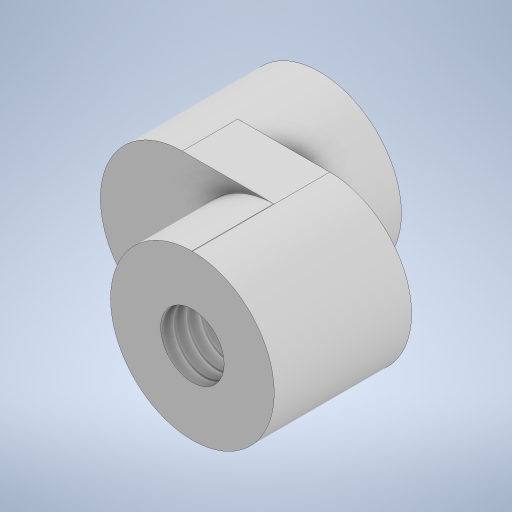
# Autodesk Inventor part: PC104_EM-113 standoff_3.57
Saved by Autodesk Inventor 2024 (Build 280153000, 153)
## iProperties
Created: 2023-04-19
Part Number: PC104_EM-113 standoff_3.57
Material: Generic
Document SubType Name: Modeling
Designer: Owner
Density: 1 g/cm^3
Appearance: Default
Author: Owner
Autodesk Inventor part; units mm, degrees
ref_plane "YZ Plane" through (0, 0, 0) normal (1, 0, 0) x (0, 1, 0)
ref_plane "XZ Plane" through (0, 0, 0) normal (0, 1, 0) x (-1, 0, 0)
ref_plane "XY Plane" through (0, 0, 0) normal (0, 0, 1) x (1, 0, 0)
sketch "Sketch2" plane through (0, 0, 0) normal (0, 0, 1) x (1, 0, 0)
  arc A0 (3.57, -3.175) -> (3.57, 3.175) centre (3.57, 0) ccw
  arc A1 (0, 3.175) -> (0, -3.175) centre (0, 0) ccw
  line L0 (0, 3.175) -> (3.57, 3.175)
  line L1 (0, -3.175) -> (3.57, -3.175)
  dimension "d14" = 6.35
  dimension "d15" = 6.35
  dimension "d16" = 0
  dimension "d17" = 0
  dimension "d18" = 3.57
  dimension "d19" = 0
  constraints: 4 end point, 4 point on circle, 4 tangent, 2 centre point
  measures "d14" diameter of A0
  measures "d15" diameter of A1
  measures "d16" distance of A1.centre point (0, 0)
  measures "d17" distance of A1.centre point (0, 0)
  measures "d18" distance of A0.centre point (0, 0)
  measures "d19" vertical distance of A0.centre point (0, 0)
extrude "Extrusion2" add sketch "Sketch2" along normal blind 8.509
sketch "Sketch3" plane through (0, 0, 8.509) normal (0, 0, 1) x (1, 0, 0)
  point P0 (0, 0)
  point P1 (3.57, 0)
  dimension "d22" = 3.57
  dimension "d23" = 0
  measures "d22" distance of point (3.57, 0) point (0, 0)
  measures "d23" vertical distance of point (3.57, 0) point (0, 0)
hole "Hole1" at (3.57, 0, 8.509) direction (0, 0, -1) diameter 2.459 depth 3.81 tip angle 118 thread size "M3x0.5" class "6H" standard "ISO Metric profile"
sketch "Sketch4" plane through (0, 0, 0) normal (0, 0, -1) x (-1, 0, 0)
  point P0 (0, 0)
hole "Hole2" at (0, 0, 0) direction (0, 0, 1) diameter 2.459 depth 3.81 tip angle 118 thread size "M3x0.5" class "6H" standard "ISO Metric profile"
sketch "Sketch5" plane through (0, 0, 0) normal (0, 0, -1) x (-1, 0, 0)
  arc A0 (-3.57, 3.175) -> (-3.57, -3.175) centre (-3.57, 0) ccw
  arc A1 (0, 3.175) -> (0, -3.175) centre (0, 0) ccw
  line L0 (0, 3.175) -> (-3.57, 3.175)
  arc A2 (0, -3.175) -> (0, 3.175) centre (0, 0) ccw projected
  line L1 (0, -3.175) -> (-3.57, -3.175)
  dimension "d42" = 3.57
  constraints: 4 end point, 4 point on circle, 3 tangent, 2 centre point, 2 coincident
  measures "d42" distance of A0.centre point (0, 0)
extrude "Extrusion3" cut sketch "Sketch5" against normal blind 3.175 from surface at 0 contours L0 A1 L1 A0
sketch "Sketch6" plane through (0, 0, 8.509) normal (0, 0, 1) x (1, 0, 0)
  arc A0 (3.5699, 3.1751) -> (3.5474, -3.175) centre (3.57, 0) ccw
  line L0 (3.5699, 3.1751) -> (-0.0001, 3.175)
  line L1 (0, -3.175) -> (3.57, -3.175) projected
  line L2 (3.5474, -3.175) -> (0, -3.175)
  arc A1 (-0.0001, 3.175) -> (0, -3.175) centre (0, 0) ccw
  dimension "d43" = 3.57
  constraints: 4 end point, 4 point on circle, 3 tangent, 2 centre point, 2 coincident, 2 point on line, 1 collinear
  measures "d43" distance of A0.centre point (0, 0)
extrude "Extrusion4" cut sketch "Sketch6" against normal blind 3.175
body "Solid2"
